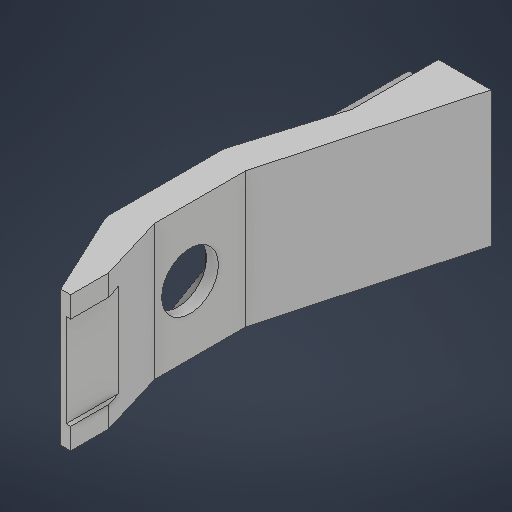
# Autodesk Inventor part: CLAMP
Saved by Autodesk Inventor 2026.2 (Build 302298000, 298)
## iProperties
Created: 2026-02-12
Part Number: CLAMP
Material: Generic
Document SubType Name: Modeling
Designer: mumin
Density: 1 g/cm^3
Appearance: Default
Author: mumin
Autodesk Inventor part; units mm, degrees
ref_plane "YZ Plane" through (0, 0, 0) normal (1, 0, 0) x (0, 1, 0)
ref_plane "XZ Plane" through (0, 0, 0) normal (0, 1, 0) x (-1, 0, 0)
ref_plane "XY Plane" through (0, 0, 0) normal (0, 0, 1) x (1, 0, 0)
sketch "Sketch1" plane through (0, 0, 0) normal (0, 1, 0) x (-1, 0, 0)
  line L0 (5.15, 19.25) -> (5.15, 15.05)
  line L1 (5.15, 15.05) -> (7.35, 7.75)
  line L2 (7.35, 7.75) -> (7.35, -2.35)
  line L3 (7.35, -2.35) -> (4.35, -13.35)
  line L4 (4.35, -23.75) -> (7.35, -23.75)
  line L5 (7.35, -23.75) -> (7.35, -14.1682)
  line L6 (7.35, -14.1682) -> (10.6664, -3.2545)
  line L7 (10.6664, -3.2545) -> (10.6664, 9.8102)
  line L8 (10.6664, 9.8102) -> (6.25, 19.25)
  line L9 (6.25, 19.25) -> (5.15, 19.25)
  line L10 (4.35, -13.35) -> (3.8238, -15.2795)
  line L11 (3.8238, -15.2795) -> (1.5136, -23.75)
  line L12 (1.5136, -23.75) -> (4.35, -23.75)
  point P0 (0, 0)
  dimension "d21" = 2
  constraints: 26 end point, 5 point on line, 3 parallel, 1 horizontal, 1 vertical
  measures "d21" distance of L3.end L10.end
extrude "Extrusion1" add sketch "Sketch1" along normal mid plane 15
sketch "Sketch2" plane through (-10.6664, -7.5, 9.8102) normal (-1, 0, 0) x (0, 0, 1)
  line L0 (0, 0) -> (0, 15) projected
  line L1 (-1, 4.6132) -> (-6, 1.7265)
  line L2 (-6, 1.7265) -> (-11, 4.6132)
  line L3 (-11, 4.6132) -> (-11, 10.3868)
  line L4 (-11, 10.3868) -> (-6, 13.2735)
  line L5 (-6, 13.2735) -> (-1, 10.3868)
  line L6 (-1, 10.3868) -> (-1, 4.6132)
  circle A0 centre (-6, 7.5) radius 3.15
  point P0 (-1, 7.5)
  dimension "d16" = 6.3
  constraints: 12 end point, 1 centre point, 1 coincident, 1 midpoint, 13 other
  measures "d16" diameter of A0
extrude "Extrusion3" cut sketch "Sketch2" against normal blind 2 contours L1 L2 L3 L4 L5 L6 | A0
extrude "Extrusion4" cut sketch "Sketch2" against normal through all contours A0
sketch "Sketch4" plane through (-6.25, 7.5, 19.25) normal (0, 0, 1) x (1, 0, 0)
  line L0 (0.6, -12.65) -> (1.6, -12.65)
  line L1 (1.6, -12.65) -> (1.6, -2.35)
  line L2 (1.6, -2.35) -> (0.6, -2.35)
  line L3 (0.6, -2.35) -> (0.6, -12.65)
  line L4 (1.1, -15) -> (1.1, 0) projected
  line L5 (0.6, -12.65) -> (1.6, -2.35) construction
  line L6 (1.6, -12.65) -> (0.6, -2.35) construction
  point P0 (6.25, -7.5)
  point P1 (1.1, -7.5)
  dimension "d22" = 1
  dimension "d23" = 10.3
  constraints: 12 end point, 3 midpoint, 2 parallel, 1 horizontal, 1 perpendicular
  measures "d22" distance of L2.end L1.end
  measures "d23" distance of L1.end L0.end
extrude "Extrusion5" cut sketch "Sketch4" against normal blind 10
sketch "Sketch5" plane through (-1.5136, 7.5, -23.75) normal (0, 0, -1) x (-1, 0, 0)
  line L0 (0, -15) -> (0, 0) projected
  line L1 (0, -7.5) -> (9.1528, -7.5)
  line L2 (2.5199, -2.75) -> (9.1528, -2.75)
  line L3 (9.1528, -2.75) -> (9.1528, -4.75)
  line L4 (9.1528, -4.75) -> (2.5199, -4.75)
  line L5 (2.5199, -4.75) -> (2.5199, -2.75)
  line L6 (5.8364, -15) -> (5.8364, 0) projected
  line L7 (2.5199, -2.75) -> (9.1528, -4.75) construction
  line L8 (9.1528, -2.75) -> (2.5199, -4.75) construction
  line L9 (2.5199, -12.25) -> (9.1528, -12.25)
  line L10 (9.1528, -12.25) -> (9.1528, -10.25)
  line L11 (9.1528, -10.25) -> (2.5199, -10.25)
  line L12 (2.5199, -10.25) -> (2.5199, -12.25)
  line L13 (2.5199, -12.25) -> (9.1528, -10.25) construction
  line L14 (9.1528, -12.25) -> (2.5199, -10.25) construction
  point P0 (-1.5136, -7.5)
  point P1 (5.8364, -3.75)
  point P2 (5.8364, -2.75)
  point P3 (5.8364, -4.75)
  point P4 (5.8364, -10.25)
  point P5 (5.8364, -12.25)
  dimension "d26" = 2
  dimension "d27" = 3.75
  constraints: 26 end point, 4 symmetric about line, 3 midpoint, 2 parallel, 1 horizontal, 1 perpendicular, 1 point on line
  measures "d26" distance of L4.end L2.start
  measures "d27" distance from line of L1 point (5.836, -3.75)
extrude "Extrusion6" add sketch "Sketch5" against normal blind 21 contours L2 L3 L4 L6 | L6 L11 L10 L9
body "Solid1"
